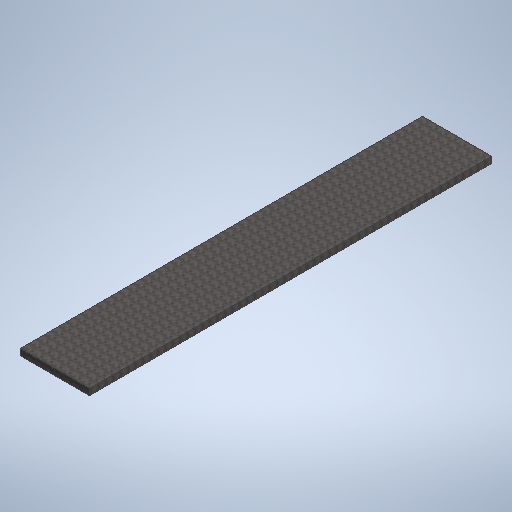
# Autodesk Inventor part: Concrete Walkway
Saved by Autodesk Inventor 2025 (Build 290162000, 162)
## iProperties
Created: 2024-06-26
Part Number: Concrete Walkway
Material: Concrete
Document SubType Name: Modeling
Designer: track
Density: 2.40731 g/cm^3
Appearance: Exposed Aggregate - Coarse
Author: track
Autodesk Inventor part; units mm, degrees
ref_plane "YZ Plane" through (0, 0, 0) normal (1, 0, 0) x (0, 1, 0)
ref_plane "XZ Plane" through (0, 0, 0) normal (0, 1, 0) x (-1, 0, 0)
ref_plane "XY Plane" through (0, 0, 0) normal (0, 0, 1) x (1, 0, 0)
sketch "Sketch1" plane through (0, 0, 0) normal (0, 0, 1) x (1, 0, 0)
  line L0 (838.2, -76.2) -> (-838.2, -76.2)
  line L1 (-838.2, -76.2) -> (-838.2, 76.2)
  line L2 (-838.2, 76.2) -> (838.2, 76.2)
  line L3 (838.2, 76.2) -> (838.2, -76.2)
  line L4 (838.2, -76.2) -> (-838.2, 76.2) construction
  line L5 (-838.2, -76.2) -> (838.2, 76.2) construction
  point P0 (0, 0)
  dimension "d0" = 152.4
  dimension "d1" = 1676.4
  constraints: 12 end point, 2 midpoint, 2 parallel, 1 horizontal, 1 perpendicular
  measures "d0" distance of L0.end L1.end
  measures "d1" distance of L1.end L2.end
extrude "Extrusion1" add sketch "Sketch1" against normal blind 9753.6
body "Solid1"
